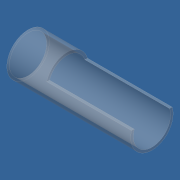
# Autodesk Inventor part: S1702_tubeexterne
Saved by Autodesk Inventor 2015 SP2 (Build 190223200, 223)
## iProperties
Created: 2017-10-26
Part Number: S1702_tubeexterne
Material: Plastique PMMA
Document SubType Name: Modeling
Designer: Benoit.CURCHOD2
Density: 1.188 g/cm^3
Appearance: Transparent - Clair
Project: S1702_circuit_voiture
Description: Tube Externe
Authority: Ø50x146
Mass: 55.5861 g
Surface Area: 327.081 cm^2
Volume: 46.7896 cm^3
Author: Benoit.CURCHOD2
Autodesk Inventor part; units mm, degrees
ref_plane "YZ Plane" through (0, 0, 0) normal (1, 0, 0) x (0, 1, 0)
ref_plane "XZ Plane" through (0, 0, 0) normal (0, 1, 0) x (-1, 0, 0)
ref_plane "XY Plane" through (0, 0, 0) normal (0, 0, 1) x (1, 0, 0)
sketch "Esquisse1" plane through (0, 0, 0) normal (0, 0, 1) x (1, 0, 0)
  line L0 (0, 25) -> (146, 25)
  line L1 (146, 25) -> (146, 22)
  line L2 (146, 22) -> (0, 22)
  line L3 (0, 22) -> (0, 25)
  line L4 (-10.0826, 0) -> (43.679, 0)
  line L5 (-41.2991, 0) -> (177.2165, 0) projected
  line L6 (0, -5) -> (0, 30) projected
  point P0 (0, 0)
  dimension "d0" = 3
  dimension "d1" = 50
  dimension "d2" = 146
  constraints: 10 end point, 3 perpendicular, 2 collinear, 2 horizontal
  measures "d0" distance of L0.end L1.end
  measures "d1" diameter of L0 L4
  measures "d2" distance of L0.start L0.end
revolve "Révolution1" add sketch "Esquisse1" angle 360 about axis through (-10.0826, 0, 0) along (1, 0, 0)
sketch "Esquisse5" plane through (146, 0, 0) normal (1, 0, 0) x (0, 0, -1)
  line L0 (-35, 0) -> (35, 0) construction
  circle A0 centre (0, 0) radius 22 construction
  circle A1 centre (0, 0) radius 25 construction
  line L1 (-25, -21.6089) -> (-25, 34.5668) construction
  line L2 (-22, -18.8661) -> (-22, 30.8732) construction
  line L3 (-7, -26.0436) -> (-7, 26.1117) construction
  arc A2 (0, 22) -> (0, 22) centre (0, 0) ccw projected
  arc A3 (-7, 20.8567) -> (-7, -20.8567) centre (0, 0) ccw
  arc A4 (0, 25) -> (0, 25) centre (0, 0) ccw projected
  arc A5 (0, 25) -> (0, 25) centre (0, 0) ccw projected
  arc A6 (-7, 24) -> (-7, -24) centre (0, 0) ccw
  line L4 (-7, -24) -> (-7, -20.8567)
  line L5 (-7, 20.8567) -> (-7, 24)
  dimension "d31" = 15
  constraints: 10 end point, 8 point on circle, 4 point on line, 3 vertical, 2 centre point, 2 collinear, 2 concentric, 2 tangent
  measures "d31" distance between parallel lines of L3 L2
extrude "Extrusion5" cut sketch "Esquisse5" against normal blind 100 contours A2 L4 A4 L5 picked at (-22.7161, 2.7828)
